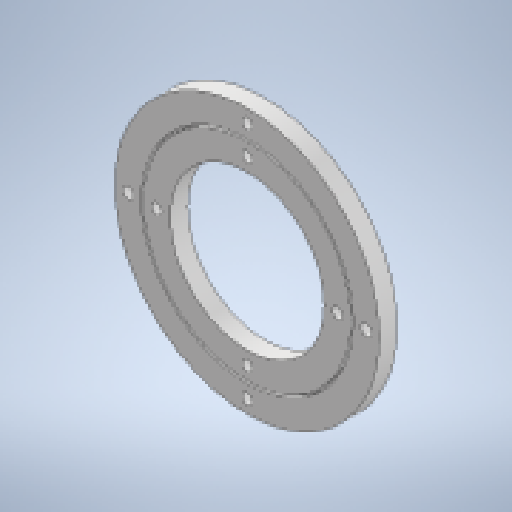
# Autodesk Inventor part: arm bearing
Saved by Autodesk Inventor 2025 (Build 290162000, 162)
## iProperties
Created: 2025-04-03
Part Number: arm bearing
Material: 一般
Document SubType Name: Modeling
Designer: gavin
Density: 1 g/cm^3
Appearance: 預設
Author: gavin
Autodesk Inventor part; units mm, degrees
ref_plane "YZ Plane" through (0, 0, 0) normal (1, 0, 0) x (0, 1, 0)
ref_plane "XZ Plane" through (0, 0, 0) normal (0, 1, 0) x (-1, 0, 0)
ref_plane "XY Plane" through (0, 0, 0) normal (0, 0, 1) x (1, 0, 0)
sketch "草圖1" plane through (0, 0, 0) normal (0, 0, 1) x (1, 0, 0)
  circle A0 centre (0, 0) radius 60
  circle A1 centre (0, 0) radius 35
  dimension "d0" = 120
  dimension "d4" = 70
  constraints: 2 centre point, 1 coincident
  measures "d0" diameter of A0
  measures "d4" diameter of A1
extrude "擠出1" add sketch "草圖1" along normal blind 8
sketch "草圖2" plane through (0, 0, 8) normal (0, 0, 1) x (1, 0, 0)
  circle A0 centre (0, 0) radius 60 projected
  circle A1 centre (0, 0) radius 35 projected
  circle A2 centre (0, 0) radius 48
  circle A3 centre (0, 0) radius 47
  dimension "d7" = 12
  dimension "d8" = 12
  constraints: 2 centre point
  measures "d7" radial gap between concentric circles of A0 A2
  measures "d8" radial gap between concentric circles of A1 A3
extrude "擠出2" cut sketch "草圖2" against normal blind 2 contours A2
sketch "草圖3" plane through (0, 0, 0) normal (0, 0, -1) x (-1, 0, 0)
  circle A0 centre (0, 0) radius 48 projected
  circle A1 centre (0, 0) radius 47 projected
  circle A2 centre (0, 0) radius 35 projected
  circle A3 centre (0, 0) radius 60 projected
extrude "擠出3" cut sketch "草圖3" against normal blind 2 contours A0
sketch "草圖4" plane through (0, 0, 8) normal (0, 0, 1) x (1, 0, 0)
  circle A0 centre (0, 0) radius 41 construction
  circle A1 centre (0, -41) radius 2.5
  circle A2 centre (0, 0) radius 41 construction
  circle A3 centre (41, 0) radius 2.5
  circle A4 centre (0, 0) radius 41 construction
  circle A5 centre (0, 41) radius 2.5
  circle A6 centre (0, 0) radius 41 construction
  circle A7 centre (-41, 0) radius 2.5
  circle A8 centre (0, 0) radius 54 construction
  circle A9 centre (0, -54) radius 2.5
  circle A10 centre (54, 0) radius 2.5
  circle A11 centre (0, 54) radius 2.5
  circle A12 centre (-54, 0) radius 2.5
  dimension "d13" = 82
  dimension "d19" = 108
  dimension "d14" = 5
  dimension "d17" = 360
  dimension "d20" = 5
  dimension "d23" = 360
  constraints: 8 centre point, 3 vertical alignment, 2 coincident, 2 horizontal alignment, 36 other
  measures "d14" diameter of A1
  measures "d20" diameter of A9
extrude "擠出4" cut sketch "草圖4" against normal through all
